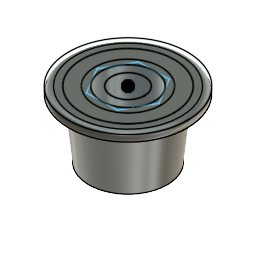
ShoeStand (Autodesk Fusion 360 design; units mm, degrees)
Autodesk Fusion 360 part; units mm, degrees
sketch "Sketch1" plane through (0, 0, 0) normal (0, 0, 1) x (1, 0, 0)
  circle A0 centre (0, 0) radius 9
  circle A1 centre (0, 0) radius 4
  line L0 (4.618, 0.0854) -> (2.235, 4.042)
  line L1 (2.235, 4.042) -> (-2.383, 3.9566)
  line L2 (-2.383, 3.9566) -> (-4.618, -0.0854)
  line L3 (-4.618, -0.0854) -> (-2.235, -4.042)
  line L4 (-2.235, -4.042) -> (2.383, -3.9566)
  line L5 (2.383, -3.9566) -> (4.618, 0.0854)
  circle A2 centre (0, 0) radius 7
  circle A3 centre (0, 0) radius 5
  circle A4 centre (0, 0) radius 2.5
  dimension "d1" = 18
  dimension "d2" = 8
  dimension "d3" = 14
  dimension "d10" = 10
  dimension "d11" = 5
  constraint coincident A0.centre A1.centre
  constraint concentric A0 A1
  constraint concentric A1 A2
  constraint concentric A1 A3
  measures "d1" diameter of A0
  measures "d2" diameter of A1
  measures "d3" diameter of A2
  measures "d10" diameter of A3
  measures "d11" diameter of A4
extrude "Extrude2" add sketch "Sketch1" against normal blind 10 draft -6 contours A1 | A1 L0 L5 | A1 L0 L1 | A1 L4 L5 | A1 L1 L2 | A1 L3 L4 | A1 L2 L3 | A2 | A3 makes body 1
extrude "Extrude3" add sketch "Sketch1" against normal blind 1 contours A0 makes body 2
extrude "Extrude4" add sketch "Sketch1" along normal blind 1 from surface at -11 contours A1 | A1 L0 L5 | A1 L0 L1 | A1 L4 L5 | A1 L1 L2 | A1 L3 L4 | A1 L2 L3 bodies 1
fillet "Fillet1" radius 1 1 edges at (-8.3909, -3.2545, 0) on bodies 2
extrude "Extrude5" cut sketch "Sketch1" against normal blind 9 contours A1 bodies 1
